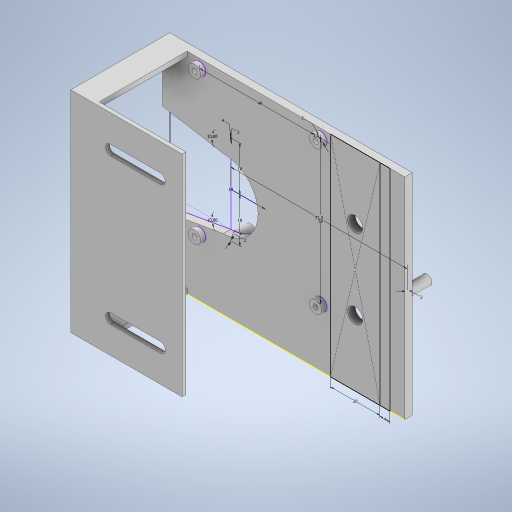
# Autodesk Inventor part: RP4_LidarHolderv3
Saved by Autodesk Inventor 2024 (Build 280153000, 153)
## iProperties
Created: 2025-05-21
Part Number: RP4_LidarHolderv3
Material: Ogólny
Document SubType Name: Modeling
Designer: Victoria
Density: 1 g/cm^3
Appearance: Domyślna
Author: Victoria
Autodesk Inventor part; units mm, degrees
ref_plane "YZ Plane" through (0, 0, 0) normal (1, 0, 0) x (0, 1, 0)
ref_plane "XZ Plane" through (0, 0, 0) normal (0, 1, 0) x (-1, 0, 0)
ref_plane "XY Plane" through (0, 0, 0) normal (0, 0, 1) x (1, 0, 0)
sketch "Szkic1" plane through (0, 0, 0) normal (0, 0, 1) x (1, 0, 0)
  circle A0 centre (0, 16) radius 3
  circle A1 centre (0, -16) radius 3
  line L0 (0, 0) -> (20, 0)
  line L1 (20, 0) -> (20, -42.5)
  line L2 (20, 0) -> (20, 42.5)
  line L3 (20, 0) -> (62.5, 0) construction
  line L4 (20, 42.5) -> (-78, 42.5)
  line L5 (-78, 42.5) -> (-78, -42.5)
  line L6 (-78, -42.5) -> (20, -42.5)
  dimension "d0" = 6
  dimension "d1" = 6
  dimension "d5" = 20
  dimension "d6" = 42.5
  dimension "d7" = 42.5
  dimension "d8" = 90
  dimension "d9" = 98
  dimension "d10" = 85
  dimension "d11" = 90
  constraints: 14 end point, 4 perpendicular, 2 centre point, 2 horizontal, 1 vertical
  measures "d0" diameter of A0
  measures "d1" diameter of A1
  measures "d5" distance of L0.start L0.end
  measures "d6" distance of L0.end L1.end
  measures "d7" distance of L0.end L2.end
  measures "d8" angle of L3 L2
  measures "d9" distance of L2.end L4.end
  measures "d10" distance of L4.end L5.end
  measures "d11" angle of L5 L4
extrude "Wyciągnięcie proste1" add sketch "Szkic1" along normal blind 3
sketch "Szkic2" plane through (0, 0, 3) normal (0, 0, 1) x (1, 0, 0)
  line L0 (-78, -42.5) -> (20, -42.5) projected
  line L1 (-10, 42.5) -> (10, 42.5)
  line L2 (10, 42.5) -> (10, -42.5)
  line L3 (10, -42.5) -> (-10, -42.5)
  line L4 (-10, -42.5) -> (-10, 42.5)
  line L5 (-10, 42.5) -> (10, -42.5) construction
  line L6 (10, 42.5) -> (-10, -42.5) construction
  circle A0 centre (-14, 39) radius 1
  circle A1 centre (-14, 39) radius 2.5
  circle A2 centre (-63, 39) radius 2.5
  circle A3 centre (-63, 39) radius 1
  circle A4 centre (-14, -19) radius 2.5
  circle A5 centre (-14, -19) radius 1
  circle A6 centre (-63, -19) radius 2.5
  circle A7 centre (-63, -19) radius 1
  line L7 (10, 42.5) -> (14, 42.5)
  line L8 (14, 42.5) -> (14, -42.5)
  line L9 (14, -42.5) -> (10, -42.5)
  line L10 (10, -42.5) -> (10, 42.5)
  point P0 (0, 0)
  dimension "d14" = 20
  dimension "d15" = 2
  dimension "d16" = 1.5
  dimension "d19" = 49
  dimension "d22" = 58
  dimension "d25" = 4
  constraints: 20 end point, 8 centre point, 4 parallel, 3 horizontal, 2 midpoint, 2 perpendicular, 2 point on line, 1 vertical, 9 other
  measures "d14" distance of L2.end L3.end
  measures "d15" diameter of A0
  measures "d16" radial gap between concentric circles of A0 A1
  measures "d19" distance of A0.centre A2.centre
  measures "d22" distance of A0.centre A4.centre
  measures "d25" distance of L8.end L9.end
extrude "Wyciągnięcie proste2" add sketch "Szkic2" along normal blind 2 contours A1 | A2 | A4 | A6
extrude "Wyciągnięcie proste3" cut sketch "Szkic2" against normal blind 3 contours A0 | A3 | A5 | A7
sketch "Szkic4" plane through (0, 0, 3) normal (0, 0, 1) x (1, 0, 0)
  line L0 (-78, 42.5) -> (-78, -42.5) projected
  line L1 (-78, -42.5) -> (-68, -42.5)
  line L2 (-68, -42.5) -> (-68, -40.5)
  line L3 (-68, -40.5) -> (-78, -40.5)
  line L4 (-78, -40.5) -> (-78, -42.5)
  line L5 (-78, 42.5) -> (-68, 42.5)
  line L6 (-68, 42.5) -> (-68, 40.5)
  line L7 (-68, 40.5) -> (-78, 40.5)
  line L8 (-78, 40.5) -> (-78, 42.5)
  point P0 (0, 0)
  dimension "d31" = 10
  dimension "d32" = 2
  dimension "d33" = 10
  dimension "d34" = 2
  constraints: 16 end point, 4 parallel, 2 horizontal, 2 perpendicular
  measures "d31" distance of L3.end L2.end
  measures "d32" distance of L2.end L1.end
  measures "d33" distance of L6.end L7.end
  measures "d34" distance of L5.end L6.end
extrude "Wyciągnięcie proste4" add sketch "Szkic4" along normal blind 37
sketch "Szkic5" plane through (0, 0, 40) normal (0, 0, 1) x (1, 0, 0)
  line L0 (-78, -42.5) -> (20, -42.5) projected
  line L1 (20, 42.5) -> (-78, 42.5) projected
  line L2 (-78, -42.5) -> (-33, -42.5)
  line L3 (-33, -42.5) -> (-33, 42.5)
  line L4 (-33, 42.5) -> (-78, 42.5)
  line L5 (-78, 42.5) -> (-78, -42.5)
  line L6 (-51.815, 0) -> (-51.815, 29.5)
  line L7 (-51.815, 29.5) -> (-51.815, -29.5)
  line L8 (-41.815, -29.5) -> (-61.815, -29.5) construction
  line L9 (-41.815, -27.5) -> (-61.815, -27.5)
  line L10 (-61.815, -31.5) -> (-41.815, -31.5)
  arc A0 (-41.815, -31.5) -> (-41.815, -27.5) centre (-41.815, -29.5) ccw
  arc A1 (-61.815, -27.5) -> (-61.815, -31.5) centre (-61.815, -29.5) ccw
  line L11 (-41.815, 29.5) -> (-61.815, 29.5) construction
  line L12 (-41.815, 31.5) -> (-61.815, 31.5)
  line L13 (-61.815, 27.5) -> (-41.815, 27.5)
  arc A2 (-41.815, 27.5) -> (-41.815, 31.5) centre (-41.815, 29.5) ccw
  arc A3 (-61.815, 31.5) -> (-61.815, 27.5) centre (-61.815, 29.5) ccw
  point P0 (0, 0)
  dimension "d37" = 45
  dimension "d38" = 29.5
  dimension "d39" = 59
  dimension "d40" = 10
  dimension "d41" = 4
  dimension "d42" = 4
  constraints: 28 end point, 8 point on circle, 8 tangent, 5 parallel, 4 centre point, 2 midpoint, 2 perpendicular, 2 point on line, 1 horizontal, 1 vertical
  measures "d37" distance of L4.end L3.end
  measures "d38" distance of L6.start L6.end
  measures "d39" distance of L6.end L7.end
  measures "d40" distance of L7.end L8.end
  measures "d41" diameter of A1
  measures "d42" diameter of A3
extrude "Wyciągnięcie proste5" add sketch "Szkic5" against normal blind 1.5
sketch "Szkic6" plane through (0, 0, 0) normal (0, 0, -1) x (-1, 0, 0)
  circle A0 centre (-18, 0) radius 2
  circle A1 centre (-18, 0) radius 1
  line L0 (-18, 0) -> (53.3, 0)
  line L1 (53.3, 0) -> (53.3, 18)
  line L2 (53.3, 0) -> (53.3, -18)
  circle A2 centre (53.3, -18) radius 1
  circle A3 centre (53.3, -18) radius 2
  circle A4 centre (53.3, 18) radius 1
  circle A5 centre (53.3, 18) radius 2
  arc A6 (53.3, 14) -> (53.3, -14) centre (53.3, 0) ccw
  line L3 (53.3, -14) -> (78, -18.3553)
  line L4 (78, 40.5) -> (78, -40.5) projected
  line L5 (53.3, -14) -> (78.381, -14) construction
  line L6 (53.3, 14) -> (78, 18.3553)
  line L7 (53.3, 14) -> (78.381, 14) construction
  line L8 (78, 18.3553) -> (78, -18.3553)
  point P0 (0, 0)
  dimension "d45" = 2
  dimension "d46" = 71.3
  dimension "d47" = 18
  dimension "d48" = 18
  dimension "d49" = 2
  dimension "d50" = 4
  dimension "d51" = 2
  dimension "d52" = 4
  dimension "d53" = 14
  dimension "d54" = 10
  dimension "d55" = 10
  constraints: 16 end point, 7 centre point, 6 coincident, 4 point on line, 3 horizontal, 2 equal length, 2 point on circle, 2 vertical, 1 collinear
  measures "d45" diameter of A1
  measures "d46" distance of L0.start L0.end
  measures "d47" distance of L0.end L1.end
  measures "d48" distance of L0.end L2.end
  measures "d49" diameter of A2
  measures "d50" diameter of A3
  measures "d51" diameter of A4
  measures "d52" diameter of A5
  measures "d53" radius of A6
  measures "d54" angle of L3 L5
  measures "d55" angle of L7 L6
extrude "Wyciągnięcie proste6" add sketch "Szkic6" along normal blind 8 contours A0 | A3 | A5
extrude "Wyciągnięcie proste7" cut sketch "Szkic6" against normal blind 3 contours A6 L1 L0 | L0 L2 A6 | L1 L6 L4 L3 L2
